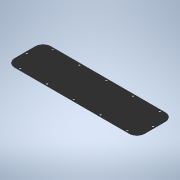
# Autodesk Inventor part: CAD_FPL_1054.000
Saved by Autodesk Inventor 2021 (Build 250183000, 183)
## iProperties
Created: 2025-08-26
Part Number: CAD_FPL_1054.000
Material: Generic
Catalog Web Link: www.cadenas.de
Description: Gland plate AX-Compact enclosures
Vendor: RITTAL
Document SubType Name: Modeling
Designer: psAdmin
Manufacturer: RITTAL
Mass: 117.298 g
Surface Area: 1587.71 cm^2
Volume: 117.298 cm^3
Density: 1 g/cm^3
Appearance: PSOLRGB-175-175-175
Category: PARTsolutions
Company: RITTAL
Title: CAD_FPL_1054.000
Author: Cadenas PARTsolutions
Comments: Compact enclosures
PSOL_IDENT_0: {$CADENAS_DATA/23d-libs/rittal/schaltschranksys/ausbauteile_cad/flanschplatten/ae_2_0_sep_fpl.prj},1
PSOL_IDENT_1: 81 {VTYP=3D},{NB=CAD_FPL_1054.000},{LINA=CAD_FPL_1054.000},{NN=Gland plate AX},{DATE=28.04.2025 21:1
PSOL_IDENT_2: 0:23},{GEOMDATE=11.04.2025 07:45:17},{VERSION=},{LINEID=340},{WBVAR=},{WBNUMERIC=}  {NB=CAD_FPL_1054
PSOL_IDENT_3: .000},{LINA=CAD_FPL_1054.000},{KT=DUMMY},{BEST=CAD_FPL_1054.000},{DETAIL=1},{VERS=7},{D=534},{E=149}
PSOL_IDENT_4: ,{BEZ1=Neues Kompaktgehäuse},{BEZ2=Stahlblech},{BEZ3=eintürig},{TUER=1},{B=600},{H=600},{T=250},{F=5
PSOL_IDENT_5: 50},{G=575},{B1=600},{B3=560.000},{B4=470.000},{B5=498.000},{BB5=0.000},{H1=600},{H3=560.000},{H4=85
PSOL_IDENT_6: .000},{H5=113.000},{HH5=4.000},{T5=93.500},{R1=31.000},{R2=8.000},{T1=250},{F1=550},{G1=575},{ST=MIN
PSOL_IDENT_7: },{VERS3=0},{CNSECLASS51=27-18-01-02},{CNSECLASS70=27-18-01-01},{CNSECLASS80=27-18-01-01},{CNSETIM40=
PSOL_IDENT_8: EC000261},{S=1.50},{W=600.000},{W1=556.000},{W2=500.000},{HH=600.000},{HH1=556.000},{HH2=550.000},{H
PSOL_IDENT_9: H3=475.000},{D1=245.100},{VERS1=1}
NB: CAD_FPL_1054.000
NN: Gland plate AX
NT: Compact enclosures
NBSYN: $BEST.
LINA: CAD_FPL_1054.000
CATALOG: Rittal
BEST: CAD_FPL_1054.000
D: 534
E: 149
SUPPLIER: RITTAL
ARTICLENO: CAD_FPL_1054.000
BOMINFO: CAD_FPL_1054.000
CREATOR: CADENAS GmbH
Autodesk Inventor part; units mm, degrees
(part 1 of 3)
sketch "Sketch_7" plane through (0, 0, 0) normal (0, 1, 0) x (1, 0, 0)
  arc A0 (-267, -42.5) -> (-235, -74.5) centre (-235, -42.5) ccw
  line L0 (-235, -74.5) -> (235, -74.5)
  arc A1 (235, -74.5) -> (267, -42.5) centre (235, -42.5) ccw
  line L1 (267, -42.5) -> (267, 42.5)
  arc A2 (267, 42.5) -> (235, 74.5) centre (235, 42.5) ccw
  line L2 (235, 74.5) -> (-235, 74.5)
  arc A3 (-235, 74.5) -> (-267, 42.5) centre (-235, 42.5) ccw
  line L3 (-267, 42.5) -> (-267, -42.5)
  circle A4 centre (259, 0) radius 3.6
  circle A5 centre (220, -66.5) radius 3.6
  circle A6 centre (220, 66.5) radius 3.6
  circle A7 centre (110, -66.5) radius 3.6
  circle A8 centre (110, 66.5) radius 3.6
  circle A9 centre (0, -66.5) radius 3.6
  circle A10 centre (0, 66.5) radius 3.6
  circle A11 centre (-110, -66.5) radius 3.6
  circle A12 centre (-110, 66.5) radius 3.6
  circle A13 centre (-220, -66.5) radius 3.6
  circle A14 centre (-220, 66.5) radius 3.6
  circle A15 centre (-259, 0) radius 3.6
  constraints: 16 centre point, 8 end point, 8 point on circle
extrude "Extrusion1" add sketch "Sketch_7" along normal blind 1.5
ref_plane "FP_XY" through (0, 0, 0) normal (0, -1, 0) x (1, 0, 0)
ref_plane "FP_YZ" through (0, 0, 0) normal (1, 0, 0) x (0, 0, 1)
ref_plane "FP_ZX" through (0, 0, 0) normal (0, 0, 1) x (0, -1, 0)
ref_plane "to_Bolt_1_XY" through (-300, 0, -300) normal (0, 1, 0) x (1, 0, 0)
ref_plane "to_Bolt_1_YZ" through (-300, 0, -300) normal (1, 0, 0) x (0, 0, -1)
ref_plane "to_Bolt_1_ZX" through (-300, 0, -300) normal (0, 0, -1) x (0, 1, 0)
ref_plane "to_Bolt_1_1_XY" through (-300, 0, -300) normal (0, 1, 0) x (1, 0, 0)
ref_plane "to_Bolt_1_1_YZ" through (-300, 0, -300) normal (1, 0, 0) x (0, 0, -1)
ref_plane "to_Bolt_1_1_ZX" through (-300, 0, -300) normal (0, 0, -1) x (0, 1, 0)
ref_plane "to_Bolt_1_10_XY" through (-278.3133, 0, -300) normal (0, 1, 0) x (1, 0, 0)
ref_plane "to_Bolt_1_10_YZ" through (-278.3133, 0, -300) normal (1, 0, 0) x (0, 0, -1)
ref_plane "to_Bolt_1_10_ZX" through (-278.3133, 0, -300) normal (0, 0, -1) x (0, 1, 0)
ref_plane "to_Bolt_1_100_XY" through (-61.4458, 0, -300) normal (0, 1, 0) x (1, 0, 0)
ref_plane "to_Bolt_1_100_YZ" through (-61.4458, 0, -300) normal (1, 0, 0) x (0, 0, -1)
ref_plane "to_Bolt_1_100_ZX" through (-61.4458, 0, -300) normal (0, 0, -1) x (0, 1, 0)
ref_plane "to_Bolt_1_101_XY" through (-59.0361, 0, -300) normal (0, 1, 0) x (1, 0, 0)
ref_plane "to_Bolt_1_101_YZ" through (-59.0361, 0, -300) normal (1, 0, 0) x (0, 0, -1)
ref_plane "to_Bolt_1_101_ZX" through (-59.0361, 0, -300) normal (0, 0, -1) x (0, 1, 0)
ref_plane "to_Bolt_1_102_XY" through (-56.6265, 0, -300) normal (0, 1, 0) x (1, 0, 0)
ref_plane "to_Bolt_1_102_YZ" through (-56.6265, 0, -300) normal (1, 0, 0) x (0, 0, -1)
ref_plane "to_Bolt_1_102_ZX" through (-56.6265, 0, -300) normal (0, 0, -1) x (0, 1, 0)
ref_plane "to_Bolt_1_103_XY" through (-54.2169, 0, -300) normal (0, 1, 0) x (1, 0, 0)
ref_plane "to_Bolt_1_103_YZ" through (-54.2169, 0, -300) normal (1, 0, 0) x (0, 0, -1)
ref_plane "to_Bolt_1_103_ZX" through (-54.2169, 0, -300) normal (0, 0, -1) x (0, 1, 0)
ref_plane "to_Bolt_1_104_XY" through (-51.8072, 0, -300) normal (0, 1, 0) x (1, 0, 0)
ref_plane "to_Bolt_1_104_YZ" through (-51.8072, 0, -300) normal (1, 0, 0) x (0, 0, -1)
ref_plane "to_Bolt_1_104_ZX" through (-51.8072, 0, -300) normal (0, 0, -1) x (0, 1, 0)
ref_plane "to_Bolt_1_105_XY" through (-49.3976, 0, -300) normal (0, 1, 0) x (1, 0, 0)
ref_plane "to_Bolt_1_105_YZ" through (-49.3976, 0, -300) normal (1, 0, 0) x (0, 0, -1)
ref_plane "to_Bolt_1_105_ZX" through (-49.3976, 0, -300) normal (0, 0, -1) x (0, 1, 0)
ref_plane "to_Bolt_1_106_XY" through (-46.988, 0, -300) normal (0, 1, 0) x (1, 0, 0)
ref_plane "to_Bolt_1_106_YZ" through (-46.988, 0, -300) normal (1, 0, 0) x (0, 0, -1)
ref_plane "to_Bolt_1_106_ZX" through (-46.988, 0, -300) normal (0, 0, -1) x (0, 1, 0)
ref_plane "to_Bolt_1_107_XY" through (-44.5783, 0, -300) normal (0, 1, 0) x (1, 0, 0)
ref_plane "to_Bolt_1_107_YZ" through (-44.5783, 0, -300) normal (1, 0, 0) x (0, 0, -1)
ref_plane "to_Bolt_1_107_ZX" through (-44.5783, 0, -300) normal (0, 0, -1) x (0, 1, 0)
ref_plane "to_Bolt_1_108_XY" through (-42.1687, 0, -300) normal (0, 1, 0) x (1, 0, 0)
ref_plane "to_Bolt_1_108_YZ" through (-42.1687, 0, -300) normal (1, 0, 0) x (0, 0, -1)
ref_plane "to_Bolt_1_108_ZX" through (-42.1687, 0, -300) normal (0, 0, -1) x (0, 1, 0)
ref_plane "to_Bolt_1_109_XY" through (-39.759, 0, -300) normal (0, 1, 0) x (1, 0, 0)
ref_plane "to_Bolt_1_109_YZ" through (-39.759, 0, -300) normal (1, 0, 0) x (0, 0, -1)
ref_plane "to_Bolt_1_109_ZX" through (-39.759, 0, -300) normal (0, 0, -1) x (0, 1, 0)
ref_plane "to_Bolt_1_11_XY" through (-275.9036, 0, -300) normal (0, 1, 0) x (1, 0, 0)
ref_plane "to_Bolt_1_11_YZ" through (-275.9036, 0, -300) normal (1, 0, 0) x (0, 0, -1)
ref_plane "to_Bolt_1_11_ZX" through (-275.9036, 0, -300) normal (0, 0, -1) x (0, 1, 0)
ref_plane "to_Bolt_1_110_XY" through (-37.3494, 0, -300) normal (0, 1, 0) x (1, 0, 0)
ref_plane "to_Bolt_1_110_YZ" through (-37.3494, 0, -300) normal (1, 0, 0) x (0, 0, -1)
ref_plane "to_Bolt_1_110_ZX" through (-37.3494, 0, -300) normal (0, 0, -1) x (0, 1, 0)
ref_plane "to_Bolt_1_111_XY" through (-34.9398, 0, -300) normal (0, 1, 0) x (1, 0, 0)
ref_plane "to_Bolt_1_111_YZ" through (-34.9398, 0, -300) normal (1, 0, 0) x (0, 0, -1)
ref_plane "to_Bolt_1_111_ZX" through (-34.9398, 0, -300) normal (0, 0, -1) x (0, 1, 0)
ref_plane "to_Bolt_1_112_XY" through (-32.5301, 0, -300) normal (0, 1, 0) x (1, 0, 0)
ref_plane "to_Bolt_1_112_YZ" through (-32.5301, 0, -300) normal (1, 0, 0) x (0, 0, -1)
ref_plane "to_Bolt_1_112_ZX" through (-32.5301, 0, -300) normal (0, 0, -1) x (0, 1, 0)
ref_plane "to_Bolt_1_113_XY" through (-30.1205, 0, -300) normal (0, 1, 0) x (1, 0, 0)
ref_plane "to_Bolt_1_113_YZ" through (-30.1205, 0, -300) normal (1, 0, 0) x (0, 0, -1)
ref_plane "to_Bolt_1_113_ZX" through (-30.1205, 0, -300) normal (0, 0, -1) x (0, 1, 0)
ref_plane "to_Bolt_1_114_XY" through (-27.7108, 0, -300) normal (0, 1, 0) x (1, 0, 0)
ref_plane "to_Bolt_1_114_YZ" through (-27.7108, 0, -300) normal (1, 0, 0) x (0, 0, -1)
ref_plane "to_Bolt_1_114_ZX" through (-27.7108, 0, -300) normal (0, 0, -1) x (0, 1, 0)
ref_plane "to_Bolt_1_115_XY" through (-25.3012, 0, -300) normal (0, 1, 0) x (1, 0, 0)
ref_plane "to_Bolt_1_115_YZ" through (-25.3012, 0, -300) normal (1, 0, 0) x (0, 0, -1)
ref_plane "to_Bolt_1_115_ZX" through (-25.3012, 0, -300) normal (0, 0, -1) x (0, 1, 0)
ref_plane "to_Bolt_1_116_XY" through (-22.8916, 0, -300) normal (0, 1, 0) x (1, 0, 0)
ref_plane "to_Bolt_1_116_YZ" through (-22.8916, 0, -300) normal (1, 0, 0) x (0, 0, -1)
ref_plane "to_Bolt_1_116_ZX" through (-22.8916, 0, -300) normal (0, 0, -1) x (0, 1, 0)
ref_plane "to_Bolt_1_117_XY" through (-20.4819, 0, -300) normal (0, 1, 0) x (1, 0, 0)
ref_plane "to_Bolt_1_117_YZ" through (-20.4819, 0, -300) normal (1, 0, 0) x (0, 0, -1)
ref_plane "to_Bolt_1_117_ZX" through (-20.4819, 0, -300) normal (0, 0, -1) x (0, 1, 0)
ref_plane "to_Bolt_1_118_XY" through (-18.0723, 0, -300) normal (0, 1, 0) x (1, 0, 0)
ref_plane "to_Bolt_1_118_YZ" through (-18.0723, 0, -300) normal (1, 0, 0) x (0, 0, -1)
ref_plane "to_Bolt_1_118_ZX" through (-18.0723, 0, -300) normal (0, 0, -1) x (0, 1, 0)
ref_plane "to_Bolt_1_119_XY" through (-15.6627, 0, -300) normal (0, 1, 0) x (1, 0, 0)
ref_plane "to_Bolt_1_119_YZ" through (-15.6627, 0, -300) normal (1, 0, 0) x (0, 0, -1)
ref_plane "to_Bolt_1_119_ZX" through (-15.6627, 0, -300) normal (0, 0, -1) x (0, 1, 0)
ref_plane "to_Bolt_1_12_XY" through (-273.494, 0, -300) normal (0, 1, 0) x (1, 0, 0)
ref_plane "to_Bolt_1_12_YZ" through (-273.494, 0, -300) normal (1, 0, 0) x (0, 0, -1)
ref_plane "to_Bolt_1_12_ZX" through (-273.494, 0, -300) normal (0, 0, -1) x (0, 1, 0)
ref_plane "to_Bolt_1_120_XY" through (-13.253, 0, -300) normal (0, 1, 0) x (1, 0, 0)
ref_plane "to_Bolt_1_120_YZ" through (-13.253, 0, -300) normal (1, 0, 0) x (0, 0, -1)
ref_plane "to_Bolt_1_120_ZX" through (-13.253, 0, -300) normal (0, 0, -1) x (0, 1, 0)
ref_plane "to_Bolt_1_121_XY" through (-10.8434, 0, -300) normal (0, 1, 0) x (1, 0, 0)
ref_plane "to_Bolt_1_121_YZ" through (-10.8434, 0, -300) normal (1, 0, 0) x (0, 0, -1)
ref_plane "to_Bolt_1_121_ZX" through (-10.8434, 0, -300) normal (0, 0, -1) x (0, 1, 0)
ref_plane "to_Bolt_1_122_XY" through (-8.4337, 0, -300) normal (0, 1, 0) x (1, 0, 0)
ref_plane "to_Bolt_1_122_YZ" through (-8.4337, 0, -300) normal (1, 0, 0) x (0, 0, -1)
ref_plane "to_Bolt_1_122_ZX" through (-8.4337, 0, -300) normal (0, 0, -1) x (0, 1, 0)
ref_plane "to_Bolt_1_123_XY" through (-6.0241, 0, -300) normal (0, 1, 0) x (1, 0, 0)
ref_plane "to_Bolt_1_123_YZ" through (-6.0241, 0, -300) normal (1, 0, 0) x (0, 0, -1)
ref_plane "to_Bolt_1_123_ZX" through (-6.0241, 0, -300) normal (0, 0, -1) x (0, 1, 0)
ref_plane "to_Bolt_1_124_XY" through (-3.6145, 0, -300) normal (0, 1, 0) x (1, 0, 0)
ref_plane "to_Bolt_1_124_YZ" through (-3.6145, 0, -300) normal (1, 0, 0) x (0, 0, -1)
ref_plane "to_Bolt_1_124_ZX" through (-3.6145, 0, -300) normal (0, 0, -1) x (0, 1, 0)
ref_plane "to_Bolt_1_125_XY" through (-1.2048, 0, -300) normal (0, 1, 0) x (1, 0, 0)
ref_plane "to_Bolt_1_125_YZ" through (-1.2048, 0, -300) normal (1, 0, 0) x (0, 0, -1)
ref_plane "to_Bolt_1_125_ZX" through (-1.2048, 0, -300) normal (0, 0, -1) x (0, 1, 0)
ref_plane "to_Bolt_1_126_XY" through (1.2048, 0, -300) normal (0, 1, 0) x (1, 0, 0)
ref_plane "to_Bolt_1_126_YZ" through (1.2048, 0, -300) normal (1, 0, 0) x (0, 0, -1)
ref_plane "to_Bolt_1_126_ZX" through (1.2048, 0, -300) normal (0, 0, -1) x (0, 1, 0)
ref_plane "to_Bolt_1_127_XY" through (3.6145, 0, -300) normal (0, 1, 0) x (1, 0, 0)
ref_plane "to_Bolt_1_127_YZ" through (3.6145, 0, -300) normal (1, 0, 0) x (0, 0, -1)
ref_plane "to_Bolt_1_127_ZX" through (3.6145, 0, -300) normal (0, 0, -1) x (0, 1, 0)
ref_plane "to_Bolt_1_128_XY" through (6.0241, 0, -300) normal (0, 1, 0) x (1, 0, 0)
ref_plane "to_Bolt_1_128_YZ" through (6.0241, 0, -300) normal (1, 0, 0) x (0, 0, -1)
ref_plane "to_Bolt_1_128_ZX" through (6.0241, 0, -300) normal (0, 0, -1) x (0, 1, 0)
ref_plane "to_Bolt_1_129_XY" through (8.4337, 0, -300) normal (0, 1, 0) x (1, 0, 0)
ref_plane "to_Bolt_1_129_YZ" through (8.4337, 0, -300) normal (1, 0, 0) x (0, 0, -1)
ref_plane "to_Bolt_1_129_ZX" through (8.4337, 0, -300) normal (0, 0, -1) x (0, 1, 0)
ref_plane "to_Bolt_1_13_XY" through (-271.0843, 0, -300) normal (0, 1, 0) x (1, 0, 0)
ref_plane "to_Bolt_1_13_YZ" through (-271.0843, 0, -300) normal (1, 0, 0) x (0, 0, -1)
ref_plane "to_Bolt_1_13_ZX" through (-271.0843, 0, -300) normal (0, 0, -1) x (0, 1, 0)
ref_plane "to_Bolt_1_130_XY" through (10.8434, 0, -300) normal (0, 1, 0) x (1, 0, 0)
ref_plane "to_Bolt_1_130_YZ" through (10.8434, 0, -300) normal (1, 0, 0) x (0, 0, -1)
ref_plane "to_Bolt_1_130_ZX" through (10.8434, 0, -300) normal (0, 0, -1) x (0, 1, 0)
ref_plane "to_Bolt_1_131_XY" through (13.253, 0, -300) normal (0, 1, 0) x (1, 0, 0)
ref_plane "to_Bolt_1_131_YZ" through (13.253, 0, -300) normal (1, 0, 0) x (0, 0, -1)
ref_plane "to_Bolt_1_131_ZX" through (13.253, 0, -300) normal (0, 0, -1) x (0, 1, 0)
ref_plane "to_Bolt_1_132_XY" through (15.6627, 0, -300) normal (0, 1, 0) x (1, 0, 0)
ref_plane "to_Bolt_1_132_YZ" through (15.6627, 0, -300) normal (1, 0, 0) x (0, 0, -1)
ref_plane "to_Bolt_1_132_ZX" through (15.6627, 0, -300) normal (0, 0, -1) x (0, 1, 0)
ref_plane "to_Bolt_1_133_XY" through (18.0723, 0, -300) normal (0, 1, 0) x (1, 0, 0)
ref_plane "to_Bolt_1_133_YZ" through (18.0723, 0, -300) normal (1, 0, 0) x (0, 0, -1)
ref_plane "to_Bolt_1_133_ZX" through (18.0723, 0, -300) normal (0, 0, -1) x (0, 1, 0)
ref_plane "to_Bolt_1_134_XY" through (20.4819, 0, -300) normal (0, 1, 0) x (1, 0, 0)
ref_plane "to_Bolt_1_134_YZ" through (20.4819, 0, -300) normal (1, 0, 0) x (0, 0, -1)
ref_plane "to_Bolt_1_134_ZX" through (20.4819, 0, -300) normal (0, 0, -1) x (0, 1, 0)
ref_plane "to_Bolt_1_135_XY" through (22.8916, 0, -300) normal (0, 1, 0) x (1, 0, 0)
ref_plane "to_Bolt_1_135_YZ" through (22.8916, 0, -300) normal (1, 0, 0) x (0, 0, -1)
ref_plane "to_Bolt_1_135_ZX" through (22.8916, 0, -300) normal (0, 0, -1) x (0, 1, 0)
ref_plane "to_Bolt_1_136_XY" through (25.3012, 0, -300) normal (0, 1, 0) x (1, 0, 0)
ref_plane "to_Bolt_1_136_YZ" through (25.3012, 0, -300) normal (1, 0, 0) x (0, 0, -1)
ref_plane "to_Bolt_1_136_ZX" through (25.3012, 0, -300) normal (0, 0, -1) x (0, 1, 0)
ref_plane "to_Bolt_1_137_XY" through (27.7108, 0, -300) normal (0, 1, 0) x (1, 0, 0)
ref_plane "to_Bolt_1_137_YZ" through (27.7108, 0, -300) normal (1, 0, 0) x (0, 0, -1)
ref_plane "to_Bolt_1_137_ZX" through (27.7108, 0, -300) normal (0, 0, -1) x (0, 1, 0)
ref_plane "to_Bolt_1_138_XY" through (30.1205, 0, -300) normal (0, 1, 0) x (1, 0, 0)
ref_plane "to_Bolt_1_138_YZ" through (30.1205, 0, -300) normal (1, 0, 0) x (0, 0, -1)
ref_plane "to_Bolt_1_138_ZX" through (30.1205, 0, -300) normal (0, 0, -1) x (0, 1, 0)
ref_plane "to_Bolt_1_139_XY" through (32.5301, 0, -300) normal (0, 1, 0) x (1, 0, 0)
ref_plane "to_Bolt_1_139_YZ" through (32.5301, 0, -300) normal (1, 0, 0) x (0, 0, -1)
ref_plane "to_Bolt_1_139_ZX" through (32.5301, 0, -300) normal (0, 0, -1) x (0, 1, 0)
ref_plane "to_Bolt_1_14_XY" through (-268.6747, 0, -300) normal (0, 1, 0) x (1, 0, 0)
ref_plane "to_Bolt_1_14_YZ" through (-268.6747, 0, -300) normal (1, 0, 0) x (0, 0, -1)
ref_plane "to_Bolt_1_14_ZX" through (-268.6747, 0, -300) normal (0, 0, -1) x (0, 1, 0)
ref_plane "to_Bolt_1_140_XY" through (34.9398, 0, -300) normal (0, 1, 0) x (1, 0, 0)
ref_plane "to_Bolt_1_140_YZ" through (34.9398, 0, -300) normal (1, 0, 0) x (0, 0, -1)
ref_plane "to_Bolt_1_140_ZX" through (34.9398, 0, -300) normal (0, 0, -1) x (0, 1, 0)
ref_plane "to_Bolt_1_141_XY" through (37.3494, 0, -300) normal (0, 1, 0) x (1, 0, 0)
ref_plane "to_Bolt_1_141_YZ" through (37.3494, 0, -300) normal (1, 0, 0) x (0, 0, -1)
ref_plane "to_Bolt_1_141_ZX" through (37.3494, 0, -300) normal (0, 0, -1) x (0, 1, 0)
ref_plane "to_Bolt_1_142_XY" through (39.759, 0, -300) normal (0, 1, 0) x (1, 0, 0)
ref_plane "to_Bolt_1_142_YZ" through (39.759, 0, -300) normal (1, 0, 0) x (0, 0, -1)
ref_plane "to_Bolt_1_142_ZX" through (39.759, 0, -300) normal (0, 0, -1) x (0, 1, 0)
ref_plane "to_Bolt_1_143_XY" through (42.1687, 0, -300) normal (0, 1, 0) x (1, 0, 0)
ref_plane "to_Bolt_1_143_YZ" through (42.1687, 0, -300) normal (1, 0, 0) x (0, 0, -1)
ref_plane "to_Bolt_1_143_ZX" through (42.1687, 0, -300) normal (0, 0, -1) x (0, 1, 0)
ref_plane "to_Bolt_1_144_XY" through (44.5783, 0, -300) normal (0, 1, 0) x (1, 0, 0)
ref_plane "to_Bolt_1_144_YZ" through (44.5783, 0, -300) normal (1, 0, 0) x (0, 0, -1)
ref_plane "to_Bolt_1_144_ZX" through (44.5783, 0, -300) normal (0, 0, -1) x (0, 1, 0)
ref_plane "to_Bolt_1_145_XY" through (46.988, 0, -300) normal (0, 1, 0) x (1, 0, 0)
ref_plane "to_Bolt_1_145_YZ" through (46.988, 0, -300) normal (1, 0, 0) x (0, 0, -1)
ref_plane "to_Bolt_1_145_ZX" through (46.988, 0, -300) normal (0, 0, -1) x (0, 1, 0)
ref_plane "to_Bolt_1_146_XY" through (49.3976, 0, -300) normal (0, 1, 0) x (1, 0, 0)
ref_plane "to_Bolt_1_146_YZ" through (49.3976, 0, -300) normal (1, 0, 0) x (0, 0, -1)
ref_plane "to_Bolt_1_146_ZX" through (49.3976, 0, -300) normal (0, 0, -1) x (0, 1, 0)
ref_plane "to_Bolt_1_147_XY" through (51.8072, 0, -300) normal (0, 1, 0) x (1, 0, 0)
ref_plane "to_Bolt_1_147_YZ" through (51.8072, 0, -300) normal (1, 0, 0) x (0, 0, -1)
ref_plane "to_Bolt_1_147_ZX" through (51.8072, 0, -300) normal (0, 0, -1) x (0, 1, 0)
ref_plane "to_Bolt_1_148_XY" through (54.2169, 0, -300) normal (0, 1, 0) x (1, 0, 0)
ref_plane "to_Bolt_1_148_YZ" through (54.2169, 0, -300) normal (1, 0, 0) x (0, 0, -1)
ref_plane "to_Bolt_1_148_ZX" through (54.2169, 0, -300) normal (0, 0, -1) x (0, 1, 0)
ref_plane "to_Bolt_1_149_XY" through (56.6265, 0, -300) normal (0, 1, 0) x (1, 0, 0)
ref_plane "to_Bolt_1_149_YZ" through (56.6265, 0, -300) normal (1, 0, 0) x (0, 0, -1)
ref_plane "to_Bolt_1_149_ZX" through (56.6265, 0, -300) normal (0, 0, -1) x (0, 1, 0)
ref_plane "to_Bolt_1_15_XY" through (-266.2651, 0, -300) normal (0, 1, 0) x (1, 0, 0)
ref_plane "to_Bolt_1_15_YZ" through (-266.2651, 0, -300) normal (1, 0, 0) x (0, 0, -1)
ref_plane "to_Bolt_1_15_ZX" through (-266.2651, 0, -300) normal (0, 0, -1) x (0, 1, 0)
ref_plane "to_Bolt_1_150_XY" through (59.0361, 0, -300) normal (0, 1, 0) x (1, 0, 0)
ref_plane "to_Bolt_1_150_YZ" through (59.0361, 0, -300) normal (1, 0, 0) x (0, 0, -1)
ref_plane "to_Bolt_1_150_ZX" through (59.0361, 0, -300) normal (0, 0, -1) x (0, 1, 0)
ref_plane "to_Bolt_1_151_XY" through (61.4458, 0, -300) normal (0, 1, 0) x (1, 0, 0)
ref_plane "to_Bolt_1_151_YZ" through (61.4458, 0, -300) normal (1, 0, 0) x (0, 0, -1)
ref_plane "to_Bolt_1_151_ZX" through (61.4458, 0, -300) normal (0, 0, -1) x (0, 1, 0)
ref_plane "to_Bolt_1_152_XY" through (63.8554, 0, -300) normal (0, 1, 0) x (1, 0, 0)
ref_plane "to_Bolt_1_152_YZ" through (63.8554, 0, -300) normal (1, 0, 0) x (0, 0, -1)
ref_plane "to_Bolt_1_152_ZX" through (63.8554, 0, -300) normal (0, 0, -1) x (0, 1, 0)
ref_plane "to_Bolt_1_153_XY" through (66.2651, 0, -300) normal (0, 1, 0) x (1, 0, 0)
ref_plane "to_Bolt_1_153_YZ" through (66.2651, 0, -300) normal (1, 0, 0) x (0, 0, -1)
ref_plane "to_Bolt_1_153_ZX" through (66.2651, 0, -300) normal (0, 0, -1) x (0, 1, 0)
ref_plane "to_Bolt_1_154_XY" through (68.6747, 0, -300) normal (0, 1, 0) x (1, 0, 0)
ref_plane "to_Bolt_1_154_YZ" through (68.6747, 0, -300) normal (1, 0, 0) x (0, 0, -1)
ref_plane "to_Bolt_1_154_ZX" through (68.6747, 0, -300) normal (0, 0, -1) x (0, 1, 0)
ref_plane "to_Bolt_1_155_XY" through (71.0843, 0, -300) normal (0, 1, 0) x (1, 0, 0)
ref_plane "to_Bolt_1_155_YZ" through (71.0843, 0, -300) normal (1, 0, 0) x (0, 0, -1)
ref_plane "to_Bolt_1_155_ZX" through (71.0843, 0, -300) normal (0, 0, -1) x (0, 1, 0)
ref_plane "to_Bolt_1_156_XY" through (73.494, 0, -300) normal (0, 1, 0) x (1, 0, 0)
ref_plane "to_Bolt_1_156_YZ" through (73.494, 0, -300) normal (1, 0, 0) x (0, 0, -1)
ref_plane "to_Bolt_1_156_ZX" through (73.494, 0, -300) normal (0, 0, -1) x (0, 1, 0)
ref_plane "to_Bolt_1_157_XY" through (75.9036, 0, -300) normal (0, 1, 0) x (1, 0, 0)
ref_plane "to_Bolt_1_157_YZ" through (75.9036, 0, -300) normal (1, 0, 0) x (0, 0, -1)
ref_plane "to_Bolt_1_157_ZX" through (75.9036, 0, -300) normal (0, 0, -1) x (0, 1, 0)
ref_plane "to_Bolt_1_158_XY" through (78.3133, 0, -300) normal (0, 1, 0) x (1, 0, 0)
ref_plane "to_Bolt_1_158_YZ" through (78.3133, 0, -300) normal (1, 0, 0) x (0, 0, -1)
ref_plane "to_Bolt_1_158_ZX" through (78.3133, 0, -300) normal (0, 0, -1) x (0, 1, 0)
ref_plane "to_Bolt_1_159_XY" through (80.7229, 0, -300) normal (0, 1, 0) x (1, 0, 0)
ref_plane "to_Bolt_1_159_YZ" through (80.7229, 0, -300) normal (1, 0, 0) x (0, 0, -1)
ref_plane "to_Bolt_1_159_ZX" through (80.7229, 0, -300) normal (0, 0, -1) x (0, 1, 0)
ref_plane "to_Bolt_1_16_XY" through (-263.8554, 0, -300) normal (0, 1, 0) x (1, 0, 0)
ref_plane "to_Bolt_1_16_YZ" through (-263.8554, 0, -300) normal (1, 0, 0) x (0, 0, -1)
ref_plane "to_Bolt_1_16_ZX" through (-263.8554, 0, -300) normal (0, 0, -1) x (0, 1, 0)
ref_plane "to_Bolt_1_160_XY" through (83.1325, 0, -300) normal (0, 1, 0) x (1, 0, 0)
ref_plane "to_Bolt_1_160_YZ" through (83.1325, 0, -300) normal (1, 0, 0) x (0, 0, -1)
ref_plane "to_Bolt_1_160_ZX" through (83.1325, 0, -300) normal (0, 0, -1) x (0, 1, 0)
ref_plane "to_Bolt_1_161_XY" through (85.5422, 0, -300) normal (0, 1, 0) x (1, 0, 0)
ref_plane "to_Bolt_1_161_YZ" through (85.5422, 0, -300) normal (1, 0, 0) x (0, 0, -1)
ref_plane "to_Bolt_1_161_ZX" through (85.5422, 0, -300) normal (0, 0, -1) x (0, 1, 0)
ref_plane "to_Bolt_1_162_XY" through (87.9518, 0, -300) normal (0, 1, 0) x (1, 0, 0)
ref_plane "to_Bolt_1_162_YZ" through (87.9518, 0, -300) normal (1, 0, 0) x (0, 0, -1)
ref_plane "to_Bolt_1_162_ZX" through (87.9518, 0, -300) normal (0, 0, -1) x (0, 1, 0)
ref_plane "to_Bolt_1_163_XY" through (90.3614, 0, -300) normal (0, 1, 0) x (1, 0, 0)
ref_plane "to_Bolt_1_163_YZ" through (90.3614, 0, -300) normal (1, 0, 0) x (0, 0, -1)
ref_plane "to_Bolt_1_163_ZX" through (90.3614, 0, -300) normal (0, 0, -1) x (0, 1, 0)
ref_plane "to_Bolt_1_164_XY" through (92.7711, 0, -300) normal (0, 1, 0) x (1, 0, 0)
ref_plane "to_Bolt_1_164_YZ" through (92.7711, 0, -300) normal (1, 0, 0) x (0, 0, -1)
ref_plane "to_Bolt_1_164_ZX" through (92.7711, 0, -300) normal (0, 0, -1) x (0, 1, 0)
ref_plane "to_Bolt_1_165_XY" through (95.1807, 0, -300) normal (0, 1, 0) x (1, 0, 0)
ref_plane "to_Bolt_1_165_YZ" through (95.1807, 0, -300) normal (1, 0, 0) x (0, 0, -1)
ref_plane "to_Bolt_1_165_ZX" through (95.1807, 0, -300) normal (0, 0, -1) x (0, 1, 0)
ref_plane "to_Bolt_1_166_XY" through (97.5904, 0, -300) normal (0, 1, 0) x (1, 0, 0)
ref_plane "to_Bolt_1_166_YZ" through (97.5904, 0, -300) normal (1, 0, 0) x (0, 0, -1)
ref_plane "to_Bolt_1_166_ZX" through (97.5904, 0, -300) normal (0, 0, -1) x (0, 1, 0)
ref_plane "to_Bolt_1_167_XY" through (100, 0, -300) normal (0, 1, 0) x (1, 0, 0)
ref_plane "to_Bolt_1_167_YZ" through (100, 0, -300) normal (1, 0, 0) x (0, 0, -1)
ref_plane "to_Bolt_1_167_ZX" through (100, 0, -300) normal (0, 0, -1) x (0, 1, 0)
ref_plane "to_Bolt_1_168_XY" through (102.4096, 0, -300) normal (0, 1, 0) x (1, 0, 0)
ref_plane "to_Bolt_1_168_YZ" through (102.4096, 0, -300) normal (1, 0, 0) x (0, 0, -1)
ref_plane "to_Bolt_1_168_ZX" through (102.4096, 0, -300) normal (0, 0, -1) x (0, 1, 0)
ref_plane "to_Bolt_1_169_XY" through (104.8193, 0, -300) normal (0, 1, 0) x (1, 0, 0)
ref_plane "to_Bolt_1_169_YZ" through (104.8193, 0, -300) normal (1, 0, 0) x (0, 0, -1)
ref_plane "to_Bolt_1_169_ZX" through (104.8193, 0, -300) normal (0, 0, -1) x (0, 1, 0)
ref_plane "to_Bolt_1_17_XY" through (-261.4458, 0, -300) normal (0, 1, 0) x (1, 0, 0)
ref_plane "to_Bolt_1_17_YZ" through (-261.4458, 0, -300) normal (1, 0, 0) x (0, 0, -1)
ref_plane "to_Bolt_1_17_ZX" through (-261.4458, 0, -300) normal (0, 0, -1) x (0, 1, 0)
ref_plane "to_Bolt_1_170_XY" through (107.2289, 0, -300) normal (0, 1, 0) x (1, 0, 0)
ref_plane "to_Bolt_1_170_YZ" through (107.2289, 0, -300) normal (1, 0, 0) x (0, 0, -1)
ref_plane "to_Bolt_1_170_ZX" through (107.2289, 0, -300) normal (0, 0, -1) x (0, 1, 0)
ref_plane "to_Bolt_1_171_XY" through (109.6386, 0, -300) normal (0, 1, 0) x (1, 0, 0)
ref_plane "to_Bolt_1_171_YZ" through (109.6386, 0, -300) normal (1, 0, 0) x (0, 0, -1)
ref_plane "to_Bolt_1_171_ZX" through (109.6386, 0, -300) normal (0, 0, -1) x (0, 1, 0)
ref_plane "to_Bolt_1_172_XY" through (112.0482, 0, -300) normal (0, 1, 0) x (1, 0, 0)
ref_plane "to_Bolt_1_172_YZ" through (112.0482, 0, -300) normal (1, 0, 0) x (0, 0, -1)
ref_plane "to_Bolt_1_172_ZX" through (112.0482, 0, -300) normal (0, 0, -1) x (0, 1, 0)
ref_plane "to_Bolt_1_173_XY" through (114.4578, 0, -300) normal (0, 1, 0) x (1, 0, 0)
ref_plane "to_Bolt_1_173_YZ" through (114.4578, 0, -300) normal (1, 0, 0) x (0, 0, -1)
ref_plane "to_Bolt_1_173_ZX" through (114.4578, 0, -300) normal (0, 0, -1) x (0, 1, 0)
ref_plane "to_Bolt_1_174_XY" through (116.8675, 0, -300) normal (0, 1, 0) x (1, 0, 0)
ref_plane "to_Bolt_1_174_YZ" through (116.8675, 0, -300) normal (1, 0, 0) x (0, 0, -1)
ref_plane "to_Bolt_1_174_ZX" through (116.8675, 0, -300) normal (0, 0, -1) x (0, 1, 0)
ref_plane "to_Bolt_1_175_XY" through (119.2771, 0, -300) normal (0, 1, 0) x (1, 0, 0)
ref_plane "to_Bolt_1_175_YZ" through (119.2771, 0, -300) normal (1, 0, 0) x (0, 0, -1)
ref_plane "to_Bolt_1_175_ZX" through (119.2771, 0, -300) normal (0, 0, -1) x (0, 1, 0)
ref_plane "to_Bolt_1_176_XY" through (121.6867, 0, -300) normal (0, 1, 0) x (1, 0, 0)
ref_plane "to_Bolt_1_176_YZ" through (121.6867, 0, -300) normal (1, 0, 0) x (0, 0, -1)
ref_plane "to_Bolt_1_176_ZX" through (121.6867, 0, -300) normal (0, 0, -1) x (0, 1, 0)
ref_plane "to_Bolt_1_177_XY" through (124.0964, 0, -300) normal (0, 1, 0) x (1, 0, 0)
ref_plane "to_Bolt_1_177_YZ" through (124.0964, 0, -300) normal (1, 0, 0) x (0, 0, -1)
ref_plane "to_Bolt_1_177_ZX" through (124.0964, 0, -300) normal (0, 0, -1) x (0, 1, 0)
ref_plane "to_Bolt_1_178_XY" through (126.506, 0, -300) normal (0, 1, 0) x (1, 0, 0)
ref_plane "to_Bolt_1_178_YZ" through (126.506, 0, -300) normal (1, 0, 0) x (0, 0, -1)
ref_plane "to_Bolt_1_178_ZX" through (126.506, 0, -300) normal (0, 0, -1) x (0, 1, 0)
ref_plane "to_Bolt_1_179_XY" through (128.9157, 0, -300) normal (0, 1, 0) x (1, 0, 0)
ref_plane "to_Bolt_1_179_YZ" through (128.9157, 0, -300) normal (1, 0, 0) x (0, 0, -1)
ref_plane "to_Bolt_1_179_ZX" through (128.9157, 0, -300) normal (0, 0, -1) x (0, 1, 0)
ref_plane "to_Bolt_1_18_XY" through (-259.0361, 0, -300) normal (0, 1, 0) x (1, 0, 0)
ref_plane "to_Bolt_1_18_YZ" through (-259.0361, 0, -300) normal (1, 0, 0) x (0, 0, -1)
ref_plane "to_Bolt_1_18_ZX" through (-259.0361, 0, -300) normal (0, 0, -1) x (0, 1, 0)
ref_plane "to_Bolt_1_180_XY" through (131.3253, 0, -300) normal (0, 1, 0) x (1, 0, 0)
ref_plane "to_Bolt_1_180_YZ" through (131.3253, 0, -300) normal (1, 0, 0) x (0, 0, -1)
ref_plane "to_Bolt_1_180_ZX" through (131.3253, 0, -300) normal (0, 0, -1) x (0, 1, 0)
ref_plane "to_Bolt_1_181_XY" through (133.7349, 0, -300) normal (0, 1, 0) x (1, 0, 0)
ref_plane "to_Bolt_1_181_YZ" through (133.7349, 0, -300) normal (1, 0, 0) x (0, 0, -1)
ref_plane "to_Bolt_1_181_ZX" through (133.7349, 0, -300) normal (0, 0, -1) x (0, 1, 0)
ref_plane "to_Bolt_1_182_XY" through (136.1446, 0, -300) normal (0, 1, 0) x (1, 0, 0)
ref_plane "to_Bolt_1_182_YZ" through (136.1446, 0, -300) normal (1, 0, 0) x (0, 0, -1)
ref_plane "to_Bolt_1_182_ZX" through (136.1446, 0, -300) normal (0, 0, -1) x (0, 1, 0)
ref_plane "to_Bolt_1_183_XY" through (138.5542, 0, -300) normal (0, 1, 0) x (1, 0, 0)
ref_plane "to_Bolt_1_183_YZ" through (138.5542, 0, -300) normal (1, 0, 0) x (0, 0, -1)
ref_plane "to_Bolt_1_183_ZX" through (138.5542, 0, -300) normal (0, 0, -1) x (0, 1, 0)
ref_plane "to_Bolt_1_184_XY" through (140.9639, 0, -300) normal (0, 1, 0) x (1, 0, 0)
ref_plane "to_Bolt_1_184_YZ" through (140.9639, 0, -300) normal (1, 0, 0) x (0, 0, -1)
ref_plane "to_Bolt_1_184_ZX" through (140.9639, 0, -300) normal (0, 0, -1) x (0, 1, 0)
ref_plane "to_Bolt_1_185_XY" through (143.3735, 0, -300) normal (0, 1, 0) x (1, 0, 0)
ref_plane "to_Bolt_1_185_YZ" through (143.3735, 0, -300) normal (1, 0, 0) x (0, 0, -1)
ref_plane "to_Bolt_1_185_ZX" through (143.3735, 0, -300) normal (0, 0, -1) x (0, 1, 0)
ref_plane "to_Bolt_1_186_XY" through (145.7831, 0, -300) normal (0, 1, 0) x (1, 0, 0)
ref_plane "to_Bolt_1_186_YZ" through (145.7831, 0, -300) normal (1, 0, 0) x (0, 0, -1)
ref_plane "to_Bolt_1_186_ZX" through (145.7831, 0, -300) normal (0, 0, -1) x (0, 1, 0)
ref_plane "to_Bolt_1_187_XY" through (148.1928, 0, -300) normal (0, 1, 0) x (1, 0, 0)
ref_plane "to_Bolt_1_187_YZ" through (148.1928, 0, -300) normal (1, 0, 0) x (0, 0, -1)
ref_plane "to_Bolt_1_187_ZX" through (148.1928, 0, -300) normal (0, 0, -1) x (0, 1, 0)
ref_plane "to_Bolt_1_188_XY" through (150.6024, 0, -300) normal (0, 1, 0) x (1, 0, 0)
ref_plane "to_Bolt_1_188_YZ" through (150.6024, 0, -300) normal (1, 0, 0) x (0, 0, -1)
ref_plane "to_Bolt_1_188_ZX" through (150.6024, 0, -300) normal (0, 0, -1) x (0, 1, 0)
ref_plane "to_Bolt_1_189_XY" through (153.012, 0, -300) normal (0, 1, 0) x (1, 0, 0)
ref_plane "to_Bolt_1_189_YZ" through (153.012, 0, -300) normal (1, 0, 0) x (0, 0, -1)
ref_plane "to_Bolt_1_189_ZX" through (153.012, 0, -300) normal (0, 0, -1) x (0, 1, 0)
ref_plane "to_Bolt_1_19_XY" through (-256.6265, 0, -300) normal (0, 1, 0) x (1, 0, 0)
ref_plane "to_Bolt_1_19_YZ" through (-256.6265, 0, -300) normal (1, 0, 0) x (0, 0, -1)
ref_plane "to_Bolt_1_19_ZX" through (-256.6265, 0, -300) normal (0, 0, -1) x (0, 1, 0)
ref_plane "to_Bolt_1_190_XY" through (155.4217, 0, -300) normal (0, 1, 0) x (1, 0, 0)
ref_plane "to_Bolt_1_190_YZ" through (155.4217, 0, -300) normal (1, 0, 0) x (0, 0, -1)
ref_plane "to_Bolt_1_190_ZX" through (155.4217, 0, -300) normal (0, 0, -1) x (0, 1, 0)
ref_plane "to_Bolt_1_191_XY" through (157.8313, 0, -300) normal (0, 1, 0) x (1, 0, 0)
ref_plane "to_Bolt_1_191_YZ" through (157.8313, 0, -300) normal (1, 0, 0) x (0, 0, -1)
ref_plane "to_Bolt_1_191_ZX" through (157.8313, 0, -300) normal (0, 0, -1) x (0, 1, 0)
ref_plane "to_Bolt_1_192_XY" through (160.241, 0, -300) normal (0, 1, 0) x (1, 0, 0)
ref_plane "to_Bolt_1_192_YZ" through (160.241, 0, -300) normal (1, 0, 0) x (0, 0, -1)
ref_plane "to_Bolt_1_192_ZX" through (160.241, 0, -300) normal (0, 0, -1) x (0, 1, 0)
ref_plane "to_Bolt_1_193_XY" through (162.6506, 0, -300) normal (0, 1, 0) x (1, 0, 0)
ref_plane "to_Bolt_1_193_YZ" through (162.6506, 0, -300) normal (1, 0, 0) x (0, 0, -1)
ref_plane "to_Bolt_1_193_ZX" through (162.6506, 0, -300) normal (0, 0, -1) x (0, 1, 0)
ref_plane "to_Bolt_1_194_XY" through (165.0602, 0, -300) normal (0, 1, 0) x (1, 0, 0)
ref_plane "to_Bolt_1_194_YZ" through (165.0602, 0, -300) normal (1, 0, 0) x (0, 0, -1)
ref_plane "to_Bolt_1_194_ZX" through (165.0602, 0, -300) normal (0, 0, -1) x (0, 1, 0)
ref_plane "to_Bolt_1_195_XY" through (167.4699, 0, -300) normal (0, 1, 0) x (1, 0, 0)
ref_plane "to_Bolt_1_195_YZ" through (167.4699, 0, -300) normal (1, 0, 0) x (0, 0, -1)
ref_plane "to_Bolt_1_195_ZX" through (167.4699, 0, -300) normal (0, 0, -1) x (0, 1, 0)
ref_plane "to_Bolt_1_196_XY" through (169.8795, 0, -300) normal (0, 1, 0) x (1, 0, 0)
ref_plane "to_Bolt_1_196_YZ" through (169.8795, 0, -300) normal (1, 0, 0) x (0, 0, -1)
ref_plane "to_Bolt_1_196_ZX" through (169.8795, 0, -300) normal (0, 0, -1) x (0, 1, 0)
ref_plane "to_Bolt_1_197_XY" through (172.2892, 0, -300) normal (0, 1, 0) x (1, 0, 0)
ref_plane "to_Bolt_1_197_YZ" through (172.2892, 0, -300) normal (1, 0, 0) x (0, 0, -1)
ref_plane "to_Bolt_1_197_ZX" through (172.2892, 0, -300) normal (0, 0, -1) x (0, 1, 0)
ref_plane "to_Bolt_1_198_XY" through (174.6988, 0, -300) normal (0, 1, 0) x (1, 0, 0)
ref_plane "to_Bolt_1_198_YZ" through (174.6988, 0, -300) normal (1, 0, 0) x (0, 0, -1)
ref_plane "to_Bolt_1_198_ZX" through (174.6988, 0, -300) normal (0, 0, -1) x (0, 1, 0)
ref_plane "to_Bolt_1_199_XY" through (177.1084, 0, -300) normal (0, 1, 0) x (1, 0, 0)
ref_plane "to_Bolt_1_199_YZ" through (177.1084, 0, -300) normal (1, 0, 0) x (0, 0, -1)
ref_plane "to_Bolt_1_199_ZX" through (177.1084, 0, -300) normal (0, 0, -1) x (0, 1, 0)
ref_plane "to_Bolt_1_2_XY" through (-297.5904, 0, -300) normal (0, 1, 0) x (1, 0, 0)
ref_plane "to_Bolt_1_2_YZ" through (-297.5904, 0, -300) normal (1, 0, 0) x (0, 0, -1)
ref_plane "to_Bolt_1_2_ZX" through (-297.5904, 0, -300) normal (0, 0, -1) x (0, 1, 0)
ref_plane "to_Bolt_1_20_XY" through (-254.2169, 0, -300) normal (0, 1, 0) x (1, 0, 0)
ref_plane "to_Bolt_1_20_YZ" through (-254.2169, 0, -300) normal (1, 0, 0) x (0, 0, -1)
ref_plane "to_Bolt_1_20_ZX" through (-254.2169, 0, -300) normal (0, 0, -1) x (0, 1, 0)
ref_plane "to_Bolt_1_200_XY" through (179.5181, 0, -300) normal (0, 1, 0) x (1, 0, 0)
ref_plane "to_Bolt_1_200_YZ" through (179.5181, 0, -300) normal (1, 0, 0) x (0, 0, -1)
ref_plane "to_Bolt_1_200_ZX" through (179.5181, 0, -300) normal (0, 0, -1) x (0, 1, 0)
ref_plane "to_Bolt_1_201_XY" through (181.9277, 0, -300) normal (0, 1, 0) x (1, 0, 0)
ref_plane "to_Bolt_1_201_YZ" through (181.9277, 0, -300) normal (1, 0, 0) x (0, 0, -1)
ref_plane "to_Bolt_1_201_ZX" through (181.9277, 0, -300) normal (0, 0, -1) x (0, 1, 0)
ref_plane "to_Bolt_1_202_XY" through (184.3373, 0, -300) normal (0, 1, 0) x (1, 0, 0)
ref_plane "to_Bolt_1_202_YZ" through (184.3373, 0, -300) normal (1, 0, 0) x (0, 0, -1)
ref_plane "to_Bolt_1_202_ZX" through (184.3373, 0, -300) normal (0, 0, -1) x (0, 1, 0)
ref_plane "to_Bolt_1_203_XY" through (186.747, 0, -300) normal (0, 1, 0) x (1, 0, 0)
ref_plane "to_Bolt_1_203_YZ" through (186.747, 0, -300) normal (1, 0, 0) x (0, 0, -1)
ref_plane "to_Bolt_1_203_ZX" through (186.747, 0, -300) normal (0, 0, -1) x (0, 1, 0)
ref_plane "to_Bolt_1_204_XY" through (189.1566, 0, -300) normal (0, 1, 0) x (1, 0, 0)
ref_plane "to_Bolt_1_204_YZ" through (189.1566, 0, -300) normal (1, 0, 0) x (0, 0, -1)
ref_plane "to_Bolt_1_204_ZX" through (189.1566, 0, -300) normal (0, 0, -1) x (0, 1, 0)
ref_plane "to_Bolt_1_205_XY" through (191.5663, 0, -300) normal (0, 1, 0) x (1, 0, 0)
ref_plane "to_Bolt_1_205_YZ" through (191.5663, 0, -300) normal (1, 0, 0) x (0, 0, -1)
ref_plane "to_Bolt_1_205_ZX" through (191.5663, 0, -300) normal (0, 0, -1) x (0, 1, 0)
ref_plane "to_Bolt_1_206_XY" through (193.9759, 0, -300) normal (0, 1, 0) x (1, 0, 0)
ref_plane "to_Bolt_1_206_YZ" through (193.9759, 0, -300) normal (1, 0, 0) x (0, 0, -1)
ref_plane "to_Bolt_1_206_ZX" through (193.9759, 0, -300) normal (0, 0, -1) x (0, 1, 0)
ref_plane "to_Bolt_1_207_XY" through (196.3855, 0, -300) normal (0, 1, 0) x (1, 0, 0)
ref_plane "to_Bolt_1_207_YZ" through (196.3855, 0, -300) normal (1, 0, 0) x (0, 0, -1)
ref_plane "to_Bolt_1_207_ZX" through (196.3855, 0, -300) normal (0, 0, -1) x (0, 1, 0)
ref_plane "to_Bolt_1_208_XY" through (198.7952, 0, -300) normal (0, 1, 0) x (1, 0, 0)
ref_plane "to_Bolt_1_208_YZ" through (198.7952, 0, -300) normal (1, 0, 0) x (0, 0, -1)
ref_plane "to_Bolt_1_208_ZX" through (198.7952, 0, -300) normal (0, 0, -1) x (0, 1, 0)
ref_plane "to_Bolt_1_209_XY" through (201.2048, 0, -300) normal (0, 1, 0) x (1, 0, 0)
ref_plane "to_Bolt_1_209_YZ" through (201.2048, 0, -300) normal (1, 0, 0) x (0, 0, -1)
ref_plane "to_Bolt_1_209_ZX" through (201.2048, 0, -300) normal (0, 0, -1) x (0, 1, 0)
ref_plane "to_Bolt_1_21_XY" through (-251.8072, 0, -300) normal (0, 1, 0) x (1, 0, 0)
ref_plane "to_Bolt_1_21_YZ" through (-251.8072, 0, -300) normal (1, 0, 0) x (0, 0, -1)
ref_plane "to_Bolt_1_21_ZX" through (-251.8072, 0, -300) normal (0, 0, -1) x (0, 1, 0)
ref_plane "to_Bolt_1_210_XY" through (203.6145, 0, -300) normal (0, 1, 0) x (1, 0, 0)
ref_plane "to_Bolt_1_210_YZ" through (203.6145, 0, -300) normal (1, 0, 0) x (0, 0, -1)
ref_plane "to_Bolt_1_210_ZX" through (203.6145, 0, -300) normal (0, 0, -1) x (0, 1, 0)
ref_plane "to_Bolt_1_211_XY" through (206.0241, 0, -300) normal (0, 1, 0) x (1, 0, 0)
ref_plane "to_Bolt_1_211_YZ" through (206.0241, 0, -300) normal (1, 0, 0) x (0, 0, -1)
ref_plane "to_Bolt_1_211_ZX" through (206.0241, 0, -300) normal (0, 0, -1) x (0, 1, 0)
ref_plane "to_Bolt_1_212_XY" through (208.4337, 0, -300) normal (0, 1, 0) x (1, 0, 0)
ref_plane "to_Bolt_1_212_YZ" through (208.4337, 0, -300) normal (1, 0, 0) x (0, 0, -1)
ref_plane "to_Bolt_1_212_ZX" through (208.4337, 0, -300) normal (0, 0, -1) x (0, 1, 0)
ref_plane "to_Bolt_1_213_XY" through (210.8434, 0, -300) normal (0, 1, 0) x (1, 0, 0)
ref_plane "to_Bolt_1_213_YZ" through (210.8434, 0, -300) normal (1, 0, 0) x (0, 0, -1)
ref_plane "to_Bolt_1_213_ZX" through (210.8434, 0, -300) normal (0, 0, -1) x (0, 1, 0)
ref_plane "to_Bolt_1_214_XY" through (213.253, 0, -300) normal (0, 1, 0) x (1, 0, 0)
ref_plane "to_Bolt_1_214_YZ" through (213.253, 0, -300) normal (1, 0, 0) x (0, 0, -1)
ref_plane "to_Bolt_1_214_ZX" through (213.253, 0, -300) normal (0, 0, -1) x (0, 1, 0)
ref_plane "to_Bolt_1_215_XY" through (215.6627, 0, -300) normal (0, 1, 0) x (1, 0, 0)
ref_plane "to_Bolt_1_215_YZ" through (215.6627, 0, -300) normal (1, 0, 0) x (0, 0, -1)
ref_plane "to_Bolt_1_215_ZX" through (215.6627, 0, -300) normal (0, 0, -1) x (0, 1, 0)
ref_plane "to_Bolt_1_216_XY" through (218.0723, 0, -300) normal (0, 1, 0) x (1, 0, 0)
ref_plane "to_Bolt_1_216_YZ" through (218.0723, 0, -300) normal (1, 0, 0) x (0, 0, -1)
ref_plane "to_Bolt_1_216_ZX" through (218.0723, 0, -300) normal (0, 0, -1) x (0, 1, 0)
ref_plane "to_Bolt_1_217_XY" through (220.4819, 0, -300) normal (0, 1, 0) x (1, 0, 0)
ref_plane "to_Bolt_1_217_YZ" through (220.4819, 0, -300) normal (1, 0, 0) x (0, 0, -1)
ref_plane "to_Bolt_1_217_ZX" through (220.4819, 0, -300) normal (0, 0, -1) x (0, 1, 0)
ref_plane "to_Bolt_1_218_XY" through (222.8916, 0, -300) normal (0, 1, 0) x (1, 0, 0)
ref_plane "to_Bolt_1_218_YZ" through (222.8916, 0, -300) normal (1, 0, 0) x (0, 0, -1)
ref_plane "to_Bolt_1_218_ZX" through (222.8916, 0, -300) normal (0, 0, -1) x (0, 1, 0)
ref_plane "to_Bolt_1_219_XY" through (225.3012, 0, -300) normal (0, 1, 0) x (1, 0, 0)
ref_plane "to_Bolt_1_219_YZ" through (225.3012, 0, -300) normal (1, 0, 0) x (0, 0, -1)
ref_plane "to_Bolt_1_219_ZX" through (225.3012, 0, -300) normal (0, 0, -1) x (0, 1, 0)
ref_plane "to_Bolt_1_22_XY" through (-249.3976, 0, -300) normal (0, 1, 0) x (1, 0, 0)
ref_plane "to_Bolt_1_22_YZ" through (-249.3976, 0, -300) normal (1, 0, 0) x (0, 0, -1)
ref_plane "to_Bolt_1_22_ZX" through (-249.3976, 0, -300) normal (0, 0, -1) x (0, 1, 0)
ref_plane "to_Bolt_1_220_XY" through (227.7108, 0, -300) normal (0, 1, 0) x (1, 0, 0)
ref_plane "to_Bolt_1_220_YZ" through (227.7108, 0, -300) normal (1, 0, 0) x (0, 0, -1)
ref_plane "to_Bolt_1_220_ZX" through (227.7108, 0, -300) normal (0, 0, -1) x (0, 1, 0)
ref_plane "to_Bolt_1_221_XY" through (230.1205, 0, -300) normal (0, 1, 0) x (1, 0, 0)
ref_plane "to_Bolt_1_221_YZ" through (230.1205, 0, -300) normal (1, 0, 0) x (0, 0, -1)
ref_plane "to_Bolt_1_221_ZX" through (230.1205, 0, -300) normal (0, 0, -1) x (0, 1, 0)
ref_plane "to_Bolt_1_222_XY" through (232.5301, 0, -300) normal (0, 1, 0) x (1, 0, 0)
ref_plane "to_Bolt_1_222_YZ" through (232.5301, 0, -300) normal (1, 0, 0) x (0, 0, -1)
ref_plane "to_Bolt_1_222_ZX" through (232.5301, 0, -300) normal (0, 0, -1) x (0, 1, 0)
ref_plane "to_Bolt_1_223_XY" through (234.9398, 0, -300) normal (0, 1, 0) x (1, 0, 0)
ref_plane "to_Bolt_1_223_YZ" through (234.9398, 0, -300) normal (1, 0, 0) x (0, 0, -1)
ref_plane "to_Bolt_1_223_ZX" through (234.9398, 0, -300) normal (0, 0, -1) x (0, 1, 0)
ref_plane "to_Bolt_1_224_XY" through (237.3494, 0, -300) normal (0, 1, 0) x (1, 0, 0)
ref_plane "to_Bolt_1_224_YZ" through (237.3494, 0, -300) normal (1, 0, 0) x (0, 0, -1)
ref_plane "to_Bolt_1_224_ZX" through (237.3494, 0, -300) normal (0, 0, -1) x (0, 1, 0)
ref_plane "to_Bolt_1_225_XY" through (239.759, 0, -300) normal (0, 1, 0) x (1, 0, 0)
ref_plane "to_Bolt_1_225_YZ" through (239.759, 0, -300) normal (1, 0, 0) x (0, 0, -1)
ref_plane "to_Bolt_1_225_ZX" through (239.759, 0, -300) normal (0, 0, -1) x (0, 1, 0)
ref_plane "to_Bolt_1_226_XY" through (242.1687, 0, -300) normal (0, 1, 0) x (1, 0, 0)
ref_plane "to_Bolt_1_226_YZ" through (242.1687, 0, -300) normal (1, 0, 0) x (0, 0, -1)
ref_plane "to_Bolt_1_226_ZX" through (242.1687, 0, -300) normal (0, 0, -1) x (0, 1, 0)
ref_plane "to_Bolt_1_227_XY" through (244.5783, 0, -300) normal (0, 1, 0) x (1, 0, 0)
ref_plane "to_Bolt_1_227_YZ" through (244.5783, 0, -300) normal (1, 0, 0) x (0, 0, -1)
ref_plane "to_Bolt_1_227_ZX" through (244.5783, 0, -300) normal (0, 0, -1) x (0, 1, 0)
ref_plane "to_Bolt_1_228_XY" through (246.988, 0, -300) normal (0, 1, 0) x (1, 0, 0)
ref_plane "to_Bolt_1_228_YZ" through (246.988, 0, -300) normal (1, 0, 0) x (0, 0, -1)
ref_plane "to_Bolt_1_228_ZX" through (246.988, 0, -300) normal (0, 0, -1) x (0, 1, 0)
ref_plane "to_Bolt_1_229_XY" through (249.3976, 0, -300) normal (0, 1, 0) x (1, 0, 0)
ref_plane "to_Bolt_1_229_YZ" through (249.3976, 0, -300) normal (1, 0, 0) x (0, 0, -1)
ref_plane "to_Bolt_1_229_ZX" through (249.3976, 0, -300) normal (0, 0, -1) x (0, 1, 0)
ref_plane "to_Bolt_1_23_XY" through (-246.988, 0, -300) normal (0, 1, 0) x (1, 0, 0)
ref_plane "to_Bolt_1_23_YZ" through (-246.988, 0, -300) normal (1, 0, 0) x (0, 0, -1)
ref_plane "to_Bolt_1_23_ZX" through (-246.988, 0, -300) normal (0, 0, -1) x (0, 1, 0)
ref_plane "to_Bolt_1_230_XY" through (251.8072, 0, -300) normal (0, 1, 0) x (1, 0, 0)
ref_plane "to_Bolt_1_230_YZ" through (251.8072, 0, -300) normal (1, 0, 0) x (0, 0, -1)
ref_plane "to_Bolt_1_230_ZX" through (251.8072, 0, -300) normal (0, 0, -1) x (0, 1, 0)
ref_plane "to_Bolt_1_231_XY" through (254.2169, 0, -300) normal (0, 1, 0) x (1, 0, 0)
ref_plane "to_Bolt_1_231_YZ" through (254.2169, 0, -300) normal (1, 0, 0) x (0, 0, -1)
ref_plane "to_Bolt_1_231_ZX" through (254.2169, 0, -300) normal (0, 0, -1) x (0, 1, 0)
ref_plane "to_Bolt_1_232_XY" through (256.6265, 0, -300) normal (0, 1, 0) x (1, 0, 0)
ref_plane "to_Bolt_1_232_YZ" through (256.6265, 0, -300) normal (1, 0, 0) x (0, 0, -1)
ref_plane "to_Bolt_1_232_ZX" through (256.6265, 0, -300) normal (0, 0, -1) x (0, 1, 0)
ref_plane "to_Bolt_1_233_XY" through (259.0361, 0, -300) normal (0, 1, 0) x (1, 0, 0)
ref_plane "to_Bolt_1_233_YZ" through (259.0361, 0, -300) normal (1, 0, 0) x (0, 0, -1)
ref_plane "to_Bolt_1_233_ZX" through (259.0361, 0, -300) normal (0, 0, -1) x (0, 1, 0)
ref_plane "to_Bolt_1_234_XY" through (261.4458, 0, -300) normal (0, 1, 0) x (1, 0, 0)
ref_plane "to_Bolt_1_234_YZ" through (261.4458, 0, -300) normal (1, 0, 0) x (0, 0, -1)
ref_plane "to_Bolt_1_234_ZX" through (261.4458, 0, -300) normal (0, 0, -1) x (0, 1, 0)
ref_plane "to_Bolt_1_235_XY" through (263.8554, 0, -300) normal (0, 1, 0) x (1, 0, 0)
ref_plane "to_Bolt_1_235_YZ" through (263.8554, 0, -300) normal (1, 0, 0) x (0, 0, -1)
ref_plane "to_Bolt_1_235_ZX" through (263.8554, 0, -300) normal (0, 0, -1) x (0, 1, 0)
ref_plane "to_Bolt_1_236_XY" through (266.2651, 0, -300) normal (0, 1, 0) x (1, 0, 0)
ref_plane "to_Bolt_1_236_YZ" through (266.2651, 0, -300) normal (1, 0, 0) x (0, 0, -1)
ref_plane "to_Bolt_1_236_ZX" through (266.2651, 0, -300) normal (0, 0, -1) x (0, 1, 0)
ref_plane "to_Bolt_1_237_XY" through (268.6747, 0, -300) normal (0, 1, 0) x (1, 0, 0)
ref_plane "to_Bolt_1_237_YZ" through (268.6747, 0, -300) normal (1, 0, 0) x (0, 0, -1)
ref_plane "to_Bolt_1_237_ZX" through (268.6747, 0, -300) normal (0, 0, -1) x (0, 1, 0)
ref_plane "to_Bolt_1_238_XY" through (271.0843, 0, -300) normal (0, 1, 0) x (1, 0, 0)
ref_plane "to_Bolt_1_238_YZ" through (271.0843, 0, -300) normal (1, 0, 0) x (0, 0, -1)
ref_plane "to_Bolt_1_238_ZX" through (271.0843, 0, -300) normal (0, 0, -1) x (0, 1, 0)
ref_plane "to_Bolt_1_239_XY" through (273.494, 0, -300) normal (0, 1, 0) x (1, 0, 0)
ref_plane "to_Bolt_1_239_YZ" through (273.494, 0, -300) normal (1, 0, 0) x (0, 0, -1)
ref_plane "to_Bolt_1_239_ZX" through (273.494, 0, -300) normal (0, 0, -1) x (0, 1, 0)
ref_plane "to_Bolt_1_24_XY" through (-244.5783, 0, -300) normal (0, 1, 0) x (1, 0, 0)
ref_plane "to_Bolt_1_24_YZ" through (-244.5783, 0, -300) normal (1, 0, 0) x (0, 0, -1)
ref_plane "to_Bolt_1_24_ZX" through (-244.5783, 0, -300) normal (0, 0, -1) x (0, 1, 0)
ref_plane "to_Bolt_1_240_XY" through (275.9036, 0, -300) normal (0, 1, 0) x (1, 0, 0)
ref_plane "to_Bolt_1_240_YZ" through (275.9036, 0, -300) normal (1, 0, 0) x (0, 0, -1)
ref_plane "to_Bolt_1_240_ZX" through (275.9036, 0, -300) normal (0, 0, -1) x (0, 1, 0)
ref_plane "to_Bolt_1_241_XY" through (278.3133, 0, -300) normal (0, 1, 0) x (1, 0, 0)
ref_plane "to_Bolt_1_241_YZ" through (278.3133, 0, -300) normal (1, 0, 0) x (0, 0, -1)
ref_plane "to_Bolt_1_241_ZX" through (278.3133, 0, -300) normal (0, 0, -1) x (0, 1, 0)
ref_plane "to_Bolt_1_242_XY" through (280.7229, 0, -300) normal (0, 1, 0) x (1, 0, 0)
ref_plane "to_Bolt_1_242_YZ" through (280.7229, 0, -300) normal (1, 0, 0) x (0, 0, -1)
ref_plane "to_Bolt_1_242_ZX" through (280.7229, 0, -300) normal (0, 0, -1) x (0, 1, 0)
ref_plane "to_Bolt_1_243_XY" through (283.1325, 0, -300) normal (0, 1, 0) x (1, 0, 0)
ref_plane "to_Bolt_1_243_YZ" through (283.1325, 0, -300) normal (1, 0, 0) x (0, 0, -1)
ref_plane "to_Bolt_1_243_ZX" through (283.1325, 0, -300) normal (0, 0, -1) x (0, 1, 0)
ref_plane "to_Bolt_1_244_XY" through (285.5422, 0, -300) normal (0, 1, 0) x (1, 0, 0)
ref_plane "to_Bolt_1_244_YZ" through (285.5422, 0, -300) normal (1, 0, 0) x (0, 0, -1)
ref_plane "to_Bolt_1_244_ZX" through (285.5422, 0, -300) normal (0, 0, -1) x (0, 1, 0)
ref_plane "to_Bolt_1_245_XY" through (287.9518, 0, -300) normal (0, 1, 0) x (1, 0, 0)
ref_plane "to_Bolt_1_245_YZ" through (287.9518, 0, -300) normal (1, 0, 0) x (0, 0, -1)
ref_plane "to_Bolt_1_245_ZX" through (287.9518, 0, -300) normal (0, 0, -1) x (0, 1, 0)
ref_plane "to_Bolt_1_246_XY" through (290.3614, 0, -300) normal (0, 1, 0) x (1, 0, 0)
ref_plane "to_Bolt_1_246_YZ" through (290.3614, 0, -300) normal (1, 0, 0) x (0, 0, -1)
ref_plane "to_Bolt_1_246_ZX" through (290.3614, 0, -300) normal (0, 0, -1) x (0, 1, 0)
ref_plane "to_Bolt_1_247_XY" through (292.7711, 0, -300) normal (0, 1, 0) x (1, 0, 0)
ref_plane "to_Bolt_1_247_YZ" through (292.7711, 0, -300) normal (1, 0, 0) x (0, 0, -1)
ref_plane "to_Bolt_1_247_ZX" through (292.7711, 0, -300) normal (0, 0, -1) x (0, 1, 0)
ref_plane "to_Bolt_1_248_XY" through (295.1807, 0, -300) normal (0, 1, 0) x (1, 0, 0)
ref_plane "to_Bolt_1_248_YZ" through (295.1807, 0, -300) normal (1, 0, 0) x (0, 0, -1)
ref_plane "to_Bolt_1_248_ZX" through (295.1807, 0, -300) normal (0, 0, -1) x (0, 1, 0)
ref_plane "to_Bolt_1_249_XY" through (297.5904, 0, -300) normal (0, 1, 0) x (1, 0, 0)
ref_plane "to_Bolt_1_249_YZ" through (297.5904, 0, -300) normal (1, 0, 0) x (0, 0, -1)
ref_plane "to_Bolt_1_249_ZX" through (297.5904, 0, -300) normal (0, 0, -1) x (0, 1, 0)
ref_plane "to_Bolt_1_25_XY" through (-242.1687, 0, -300) normal (0, 1, 0) x (1, 0, 0)
ref_plane "to_Bolt_1_25_YZ" through (-242.1687, 0, -300) normal (1, 0, 0) x (0, 0, -1)
ref_plane "to_Bolt_1_25_ZX" through (-242.1687, 0, -300) normal (0, 0, -1) x (0, 1, 0)
ref_plane "to_Bolt_1_250_XY" through (300, 0, -300) normal (0, 1, 0) x (1, 0, 0)
ref_plane "to_Bolt_1_250_YZ" through (300, 0, -300) normal (1, 0, 0) x (0, 0, -1)
ref_plane "to_Bolt_1_250_ZX" through (300, 0, -300) normal (0, 0, -1) x (0, 1, 0)
ref_plane "to_Bolt_1_251_XY" through (-300, 0, 300) normal (0, 1, 0) x (1, 0, 0)
ref_plane "to_Bolt_1_251_YZ" through (-300, 0, 300) normal (1, 0, 0) x (0, 0, -1)
ref_plane "to_Bolt_1_251_ZX" through (-300, 0, 300) normal (0, 0, -1) x (0, 1, 0)
ref_plane "to_Bolt_1_252_XY" through (-297.5904, 0, 300) normal (0, 1, 0) x (1, 0, 0)
ref_plane "to_Bolt_1_252_YZ" through (-297.5904, 0, 300) normal (1, 0, 0) x (0, 0, -1)
ref_plane "to_Bolt_1_252_ZX" through (-297.5904, 0, 300) normal (0, 0, -1) x (0, 1, 0)
ref_plane "to_Bolt_1_253_XY" through (-295.1807, 0, 300) normal (0, 1, 0) x (1, 0, 0)
ref_plane "to_Bolt_1_253_YZ" through (-295.1807, 0, 300) normal (1, 0, 0) x (0, 0, -1)
ref_plane "to_Bolt_1_253_ZX" through (-295.1807, 0, 300) normal (0, 0, -1) x (0, 1, 0)
ref_plane "to_Bolt_1_254_XY" through (-292.7711, 0, 300) normal (0, 1, 0) x (1, 0, 0)
ref_plane "to_Bolt_1_254_YZ" through (-292.7711, 0, 300) normal (1, 0, 0) x (0, 0, -1)
ref_plane "to_Bolt_1_254_ZX" through (-292.7711, 0, 300) normal (0, 0, -1) x (0, 1, 0)
ref_plane "to_Bolt_1_255_XY" through (-290.3614, 0, 300) normal (0, 1, 0) x (1, 0, 0)
ref_plane "to_Bolt_1_255_YZ" through (-290.3614, 0, 300) normal (1, 0, 0) x (0, 0, -1)
ref_plane "to_Bolt_1_255_ZX" through (-290.3614, 0, 300) normal (0, 0, -1) x (0, 1, 0)
ref_plane "to_Bolt_1_256_XY" through (-287.9518, 0, 300) normal (0, 1, 0) x (1, 0, 0)
ref_plane "to_Bolt_1_256_YZ" through (-287.9518, 0, 300) normal (1, 0, 0) x (0, 0, -1)
ref_plane "to_Bolt_1_256_ZX" through (-287.9518, 0, 300) normal (0, 0, -1) x (0, 1, 0)
ref_plane "to_Bolt_1_257_XY" through (-285.5422, 0, 300) normal (0, 1, 0) x (1, 0, 0)
ref_plane "to_Bolt_1_257_YZ" through (-285.5422, 0, 300) normal (1, 0, 0) x (0, 0, -1)
ref_plane "to_Bolt_1_257_ZX" through (-285.5422, 0, 300) normal (0, 0, -1) x (0, 1, 0)
ref_plane "to_Bolt_1_258_XY" through (-283.1325, 0, 300) normal (0, 1, 0) x (1, 0, 0)
ref_plane "to_Bolt_1_258_YZ" through (-283.1325, 0, 300) normal (1, 0, 0) x (0, 0, -1)
ref_plane "to_Bolt_1_258_ZX" through (-283.1325, 0, 300) normal (0, 0, -1) x (0, 1, 0)
ref_plane "to_Bolt_1_259_XY" through (-280.7229, 0, 300) normal (0, 1, 0) x (1, 0, 0)
ref_plane "to_Bolt_1_259_YZ" through (-280.7229, 0, 300) normal (1, 0, 0) x (0, 0, -1)
ref_plane "to_Bolt_1_259_ZX" through (-280.7229, 0, 300) normal (0, 0, -1) x (0, 1, 0)
ref_plane "to_Bolt_1_26_XY" through (-239.759, 0, -300) normal (0, 1, 0) x (1, 0, 0)
ref_plane "to_Bolt_1_26_YZ" through (-239.759, 0, -300) normal (1, 0, 0) x (0, 0, -1)